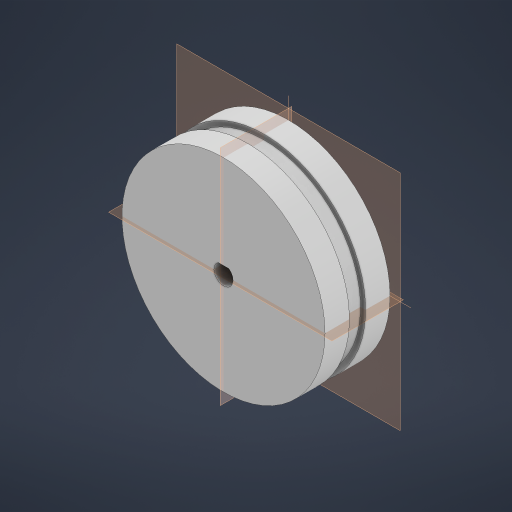
# Autodesk Inventor part: Part1
Saved by Autodesk Inventor 2024.1 (Build 281209000, 209)
## iProperties
Created: 2023-11-01
Part Number: Part1
Material: Generic
Document SubType Name: Modeling
Designer: jerem
Density: 1 g/cm^3
Appearance: Default
Author: jerem
Autodesk Inventor part; units mm, degrees
sketch "Sketch1" plane through (0, 0, 0) normal (0, 0, 1) x (1, 0, 0)
  circle A0 centre (0, 0) radius 31.75
  circle A1 centre (0, 0) radius 3
  line L0 (0, -3) -> (0, 2.5) construction
  line L1 (0, 2.5) -> (1.6583, 2.5)
  line L2 (0, 2.5) -> (-1.6583, 2.5)
  dimension "d0" = 63.5
  dimension "d1" = 6
  dimension "d2" = 5.5
  constraints: 6 end point, 3 point on circle, 2 centre point, 2 coincident, 2 horizontal, 1 vertical
  measures "d0" diameter of A0
  measures "d1" diameter of A1
  measures "d2" distance of L0.start L0.end
extrude "Extrusion1" add sketch "Sketch1" along normal blind 20.32 contours A0 | L1 L2 A1 picked at (-0.897, 2.6056)
sketch "Sketch2" plane through (0, 0, 0) normal (0, 1, 0) x (-1, 0, 0)
  line L0 (31.75, 7.62) -> (30.1625, 7.62)
  line L1 (30.1625, 7.62) -> (30.1625, 12.7)
  line L2 (30.1625, 12.7) -> (31.75, 12.7)
  line L3 (31.75, 7.62) -> (31.75, 12.7)
  line L4 (31.75, 0) -> (31.75, 7.62)
  line L5 (31.75, 20.32) -> (-31.75, 20.32) projected
  line L6 (31.75, 12.7) -> (31.75, 20.32)
  line L7 (0, -4.064) -> (0, 24.384) projected
  point P0 (0, 0)
  point P1 (31.75, 10.16)
  dimension "d5" = 5.08
  dimension "d6" = 1.5875
  dimension "d7" = 7.62
  constraints: 12 end point, 1 collinear, 1 horizontal, 1 midpoint, 1 parallel, 1 perpendicular, 1 vertical
  measures "d5" distance of L0.end L1.end
  measures "d6" distance of L0.start L0.end
  measures "d7" distance of L4.start L0.start
revolve "Revolution1" cut sketch "Sketch2" angle 360 about axis through (0, 0, -10) along (0, 0, 1)
body "Solid1"
